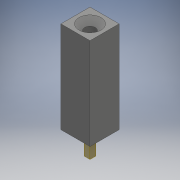
# Autodesk Inventor part: pinheader_female
Saved by Autodesk Inventor 2017 (Build 210142000, 142)
## iProperties
Created: 2017-09-13
Part Number: pinheader_female
Material: Generic
Document SubType Name: Modeling
Designer: erwin
Density: 1 g/cm^3
Appearance: Default
Author: erwin
Autodesk Inventor part; units mm, degrees
ref_plane "YZ Plane" through (0, 0, 0) normal (1, 0, 0) x (0, 1, 0)
ref_plane "Work Plane1" through (0, 0, 0) normal (0, 0, 1) x (1, 0, 0)
sketch "Sketch1" plane through (0, 0, 0) normal (0, 0, 1) x (1, 0, 0)
  circle A0 centre (3.81, 15.24) radius 0.4572 projected
  line L0 (4.06, 15.49) -> (3.56, 15.49)
  line L1 (3.56, 15.49) -> (3.56, 14.99)
  line L2 (3.56, 14.99) -> (4.06, 14.99)
  line L3 (4.06, 14.99) -> (4.06, 15.49)
  line L4 (4.06, 15.49) -> (3.56, 14.99) construction
  line L5 (3.56, 15.49) -> (4.06, 14.99) construction
  point P0 (0, 0)
  dimension "d0" = 0.5
  dimension "d1" = 0.5
  constraints: 12 end point, 2 midpoint, 2 parallel, 1 horizontal, 1 perpendicular
  measures "d0" distance of L2.end L1.end
  measures "d1" distance of L1.end L0.end
extrude "Extrusion1" add sketch "Sketch1" against normal blind 2 contours L3 L2 L1 L0
ref_plane "Work Plane2" through (0, 0, 0) normal (0, 0, 1) x (1, 0, 0)
sketch "Sketch2" plane through (0, 0, 0) normal (0, 0, 1) x (1, 0, 0)
  circle A0 centre (3.81, 15.24) radius 0.4572 projected
  line L0 (5.08, 16.51) -> (2.54, 16.51)
  line L1 (2.54, 16.51) -> (2.54, 13.97)
  line L2 (2.54, 13.97) -> (5.08, 13.97)
  line L3 (5.08, 13.97) -> (5.08, 16.51)
  line L4 (5.08, 16.51) -> (2.54, 13.97) construction
  line L5 (2.54, 16.51) -> (5.08, 13.97) construction
  point P0 (0, 0)
  dimension "d4" = 2.54
  dimension "d5" = 2.54
  constraints: 12 end point, 2 midpoint, 2 parallel, 1 horizontal, 1 perpendicular
  measures "d4" distance of L2.end L1.end
  measures "d5" distance of L1.end L0.end
extrude "Extrusion2" add sketch "Sketch2" along normal blind 8 separate body
chamfer "Chamfer1" distance 0.5 angle 45 1 edges at (3.3528, 15.24, 8)
body "Solid1"
body "Solid2"
